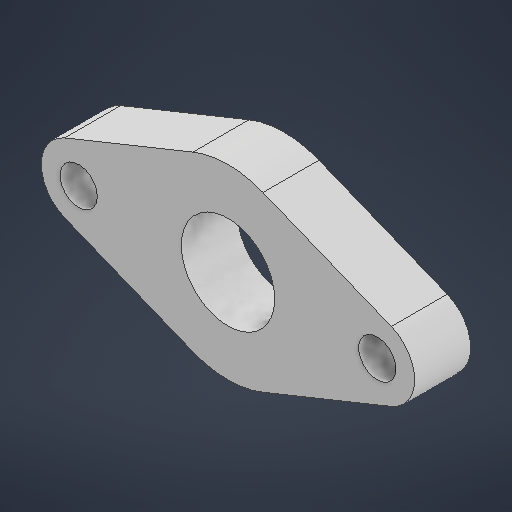
# Autodesk Inventor part: Part9
Saved by Autodesk Inventor 2026 (Build 300175050, 175E)
## iProperties
Created: 2026-03-26
Part Number: Part9
Material: Generic
Document SubType Name: Modeling
Designer: Administrator
Density: 1 g/cm^3
Appearance: Default
Author: Administrator
Autodesk Inventor part; units mm, degrees
ref_plane "YZ Plane" through (0, 0, 0) normal (1, 0, 0) x (0, 1, 0)
ref_plane "XZ Plane" through (0, 0, 0) normal (0, 1, 0) x (-1, 0, 0)
ref_plane "XY Plane" through (0, 0, 0) normal (0, 0, 1) x (1, 0, 0)
sketch "Sketch1" plane through (0, 0, 0) normal (0, 0, 1) x (1, 0, 0)
  line L0 (0, 0) -> (80, 0)
  circle A0 centre (0, 0) radius 5
  arc A1 (-3.75, 9.2702) -> (-3.75, -9.2702) centre (0, 0) ccw
  circle A2 centre (80, 0) radius 5
  arc A3 (83.75, -9.2702) -> (83.75, 9.2702) centre (80, 0) ccw
  circle A4 centre (40, 0) radius 12.5
  line L1 (-3.75, 9.2702) -> (30.625, 23.1756)
  line L2 (-3.75, -9.2702) -> (30.625, -23.1756)
  line L3 (49.375, -23.1756) -> (83.75, -9.2702)
  line L4 (106.6667, 0) -> (111.5084, 1.9586)
  line L5 (49.375, 23.1756) -> (83.75, 9.2702)
  line L6 (106.6667, 0) -> (112.4269, -2.3301)
  arc A5 (30.625, -23.1756) -> (49.375, -23.1756) centre (40, 0) ccw
  arc A6 (49.375, 23.1756) -> (30.625, 23.1756) centre (40, 0) ccw
  dimension "d0" = 80
  dimension "d1" = 20
  dimension "d2" = 10
  dimension "d4" = 25
  dimension "d5" = 20
  dimension "d6" = 10
  dimension "d7" = 40
  constraints: 14 end point, 12 tangent, 8 point on circle, 7 centre point, 5 coincident, 1 horizontal, 1 midpoint
  measures "d0" distance of L0.start L0.end
  measures "d1" diameter of A1
  measures "d2" diameter of A0
  measures "d4" diameter of A4
  measures "d5" diameter of A3
  measures "d6" diameter of A2
  measures "d7" distance of L0.end A4.centre
extrude "Extrusion1" add sketch "Sketch1" along normal mid plane 15
body "Solid1"
